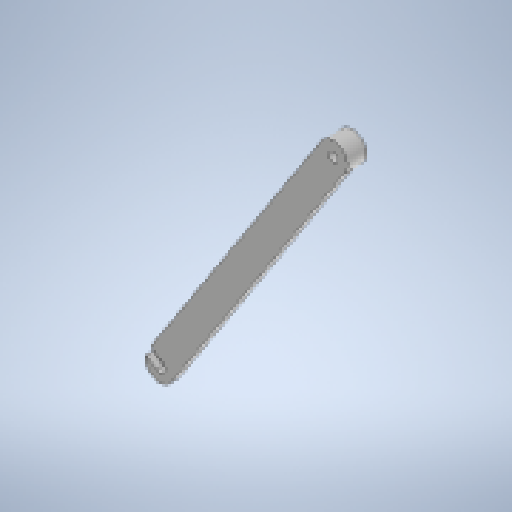
# Autodesk Inventor part: TheHandle
Saved by Autodesk Inventor 2025.1 (Build 291241000, 241)
## iProperties
Created: 2026-05-10
Part Number: TheHandle
Material: Generic
Document SubType Name: Modeling
Designer: User
Density: 1 g/cm^3
Appearance: Default
Author: User
## iProperties of the stored document TheHandle_Left_3DPrint.ipt
Created: 2026-05-12
Part Number: TheHandle_Left_3DPrint
Material: Generic
Document SubType Name: Modeling
Designer: User
Density: 1 g/cm^3
Appearance: Default
Author: User
Autodesk Inventor part; units mm, degrees
ref_plane "YZ Plane" through (0, 0, 0) normal (1, 0, 0) x (0, 1, 0)
ref_plane "XZ Plane" through (0, 0, 0) normal (0, 1, 0) x (-1, 0, 0)
ref_plane "XY Plane" through (0, 0, 0) normal (0, 0, 1) x (1, 0, 0)
sketch "Sketch1" plane through (0, 0, 0) normal (0, 0, 1) x (1, 0, 0)
  circle A0 centre (33.7394, 8.5) radius 2.5 projected
  circle A1 centre (-57.3324, -132.0207) radius 2.5 projected
  circle A2 centre (33.7394, 8.5) radius 7.5
  line L0 (40.0332, 4.421) -> (-51.0386, -136.0997)
  arc A3 (-64.7058, -130.6488) -> (-58.937, -134.5557) centre (33.7394, 8.5) ccw
  line L1 (27.4456, 12.579) -> (-61.9015, -125.2806)
  arc A4 (-64.7058, -130.6488) -> (-51.0386, -136.0997) centre (-57.3324, -132.0207) ccw
  arc A5 (-58.991, -134.5207) -> (-55.7273, -129.486) centre (-57.3324, -132.0207) ccw
  arc A6 (-61.9015, -125.2806) -> (-55.6742, -129.5204) centre (33.7394, 8.5) ccw
  point P0 (0, 0)
  dimension "d1" = 15
  constraints: 14 point on circle, 5 centre point, 4 coincident, 4 end point, 3 tangent
  measures "d1" diameter of A2
extrude "Extrusion1" add sketch "Sketch1" along normal blind 4 contours A2 | A2 L0 A4 A3 A5 A6 L1
sketch "Sketch2" plane through (0, 0, 0) normal (0, 0, -1) x (-1, 0, 0)
  circle A0 centre (-33.7394, 8.5) radius 2.5 projected
  circle A1 centre (-33.7394, 8.5) radius 2.5 projected
  circle A2 centre (-33.7394, 8.5) radius 7.5
  point P0 (0, 0)
  constraints: 1 centre point, 1 coincident
ref_plane "Work Plane1" through (-39.4645, -13.5002, -6.146) normal (0, 0, 1) x (1, 0.0000023, 0)
extrude "Extrusion2" add sketch "Sketch2" along normal up to surface (6.146 mm away)
sketch "Sketch3" plane through (0, 0, 4) normal (0, 0, 1) x (1, 0, 0)
  arc A0 (-64.7058, -130.6488) -> (-51.0386, -136.0997) centre (-57.3324, -132.0207) ccw projected
  arc A1 (-64.7058, -130.6488) -> (-58.991, -134.5207) centre (33.7394, 8.5) ccw projected
  line L0 (-51.0386, -136.0997) -> (40.0332, 4.421) projected
  line L1 (43.3899, 2.2455) -> (-47.6819, -138.2752)
  arc A2 (-66.1549, -124.6441) -> (-47.6819, -138.2752) centre (-57.3324, -132.0207) ccw
  arc A3 (-66.1549, -124.6441) -> (-56.8149, -131.1644) centre (33.7394, 8.5) ccw
  arc A4 (-58.991, -134.5207) -> (-55.7273, -129.486) centre (-57.3324, -132.0207) ccw projected
  arc A5 (-64.7058, -130.6488) -> (-58.991, -134.5207) centre (33.7394, 8.5) ccw projected
  line L2 (-58.991, -134.5207) -> (-64.7058, -130.6488)
  line L3 (-58.991, -134.5207) -> (-68.2061, -128.2773)
  line L4 (48.5795, -33.2403) -> (24.2754, 1.9668)
  line L5 (45.2876, -35.5127) -> (20.9835, -0.3056)
  point P0 (0, 0)
  point P1 (31.6873, -15.8111)
  point P2 (29.2288, -12.2498)
  point P3 (-64.7058, -130.6488)
  dimension "d9" = 4
  dimension "d10" = 4
  constraints: 10 end point, 5 point on circle, 2 centre point, 1 parallel, 1 point on line, 5 other
  measures "d9" distance between parallel lines of L0 L1
  measures "d10" distance between parallel lines of L4 L5
extrude "Extrusion3" add sketch "Sketch3" along normal mid plane 8 contours A0 L0 L5 L1 A2 L3
sketch "Sketch4" plane through (0, 0, 4) normal (0, 0, 1) x (1, 0, 0)
  line L0 (31.6873, -15.8111) -> (29.2288, -12.2498) projected
  line L1 (27.4456, 12.579) -> (-61.9015, -125.2806) projected
  line L2 (29.2288, -12.2498) -> (40.0332, 4.421) projected
  line L3 (31.6873, -15.8111) -> (-47.6819, -138.2752) projected
  line L4 (31.6873, -15.8111) -> (20.0095, 1.1054)
  line L5 (28.3955, -18.0836) -> (16.7177, -1.167)
  line L6 (-51.0386, -136.0997) -> (29.2288, -12.2498) projected
  point P0 (0, 0)
  point P1 (26.8752, -15.8813)
  point P2 (17.6559, -2.5262)
  dimension "d13" = 4
  constraints: 4 end point, 1 parallel, 1 point on line
  measures "d13" distance between parallel lines of L4 L5
extrude "Extrusion4" add sketch "Sketch4" along normal up to surface (4 mm away)
sketch "Sketch5" plane through (0, 0, 0) normal (0, 0, -1) x (-1, 0, 0)
  line L0 (51.0386, -136.0997) -> (-40.0332, 4.421)
  line L1 (-29.2288, -12.2498) -> (-31.6873, -15.8111) projected
  arc A0 (-27.4456, 12.579) -> (-40.0332, 4.421) centre (-33.7394, 8.5) ccw
  line L2 (-31.6873, -15.8111) -> (-42.9295, 11.0274)
  circle A1 centre (-33.7394, 8.5) radius 7.5 projected
  point P0 (0, 0)
  point P1 (-40.657, 5.6023)
  constraints: 4 end point, 2 point on circle, 1 centre point, 1 tangent, 6 other
extrude "Extrusion5" add sketch "Sketch5" against normal up to surface (4 mm away) contours L1 L2 A0 L0
sketch "Sketch6" plane through (33.7394, 8.5, -6.146) normal (0, 0, -1) x (-1, 0, 0)
  line L0 (106.0034, -163.8557) -> (-106.0036, -163.8552)
  line L1 (106.004, 60.4363) -> (-106.003, 60.4368)
  line L2 (0.0005, 60.4366) -> (-28.9075, 60.4367)
  line L3 (0.0005, 60.4366) -> (28.9085, 60.4365)
  circle A0 centre (0.0005, 60.4366) radius 28.908
  line L4 (0.0005, 60.4366) -> (0.0005, 100.4366)
  circle A1 centre (0.0005, 100.4366) radius 2.5
  circle A2 centre (0.0005, 100.4366) radius 7.5
  arc A3 (6.1722, -4.2608) -> (-6.1722, 4.2608) centre (0, 0) ccw
  circle A4 centre (0, 0) radius 7.5
  circle A5 centre (0, 0) radius 7.5 projected
  line L5 (7.5005, 100.4366) -> (7.5, 0)
  line L6 (-7.4995, 100.4366) -> (-7.5, 0)
  point P0 (33.7394, -8.5)
  point P1 (-7.5, 0)
  point P2 (-6.1722, 4.2608)
  point P3 (7.5, 0)
  dimension "d21" = 57.816
  dimension "d18" = 224.292
  dimension "d19" = 28.908
  dimension "d20" = 28.908
  dimension "d22" = 40
  dimension "d23" = 5
  dimension "d24" = 15
  constraints: 14 end point, 6 point on circle, 4 centre point, 4 coincident, 4 tangent, 2 point on line, 1 midpoint, 1 parallel, 1 vertical, 10 other
  measures "d18" distance between parallel lines of L0 L1
  measures "d19" distance of L2.start L2.end
  measures "d20" distance of L2.start L3.end
  measures "d22" distance of L4.start L4.end
  measures "d23" diameter of A1
  measures "d24" diameter of A2
extrude "Extrusion6" add sketch "Sketch6" against normal up to surface (10.146 mm away) contours L5 A0 L6 L1 | L1 L4 A0 L5 | A0 L4 A2 L5 | L5 A3 A4 L6 A0 | L1 L6 A0 L4 | A0 L6 A2 L4 | A2
chamfer "Chamfer1" distance 6 angle 45 3 edges at (40.3714, 4.9977, 0) (31.6126, 1.3079, 0) (26.2394, 9.6089, 0)
chamfer "Chamfer2" distance 6 angle 45 1 edges at (26.2394, 10.7178, 2)
sketch "Sketch7" plane through (0, 0, 4) normal (0, 0, 1) x (1, 0, 0)
  line L0 (45.2389, 108.9366) -> (45.2393, 24.3216)
  line L1 (41.2393, 20.3216) -> (41.2389, 108.9366)
  line L2 (45.2393, 24.3216) -> (41.2393, 20.3216)
  arc A0 (41.2389, 108.9366) -> (26.2389, 108.9366) centre (33.7389, 108.9366) ccw
  arc A1 (45.2389, 108.9366) -> (22.2389, 108.9365) centre (33.7389, 108.9366) ccw
  line L3 (22.2393, 25.7358) -> (22.2389, 108.9365)
  line L4 (26.2393, 22.1725) -> (26.2389, 108.9366)
  line L5 (22.2393, 24.3216) -> (22.2393, 25.7358)
  arc A2 (26.2393, 22.1725) -> (25.9597, 22.0154) centre (33.7394, 8.5) ccw
  arc A3 (25.9597, 22.0154) -> (25.0869, 21.474) centre (33.7394, 8.5) ccw
  line L6 (22.2393, 25.7358) -> (25.9597, 22.0154)
  point P0 (0, 0)
  constraints: 14 end point, 8 point on circle, 4 centre point, 26 other
extrude "Extrusion7" add sketch "Sketch7" along normal mid plane 10
chamfer "Chamfer3" distance 4 angle 45 3 edges at (33.7389, 116.4366, -1) (41.2391, 64.6291, -1) (26.2391, 65.5545, -1)
sketch "Sketch8" plane through (0, 0, 4) normal (0, 0, 1) x (1, 0, 0)
  circle A0 centre (33.7394, 8.5) radius 2.5
  line L0 (31.6873, -15.8111) -> (20.0095, 1.1054) projected
  line L1 (26.8752, -15.8813) -> (17.6559, -2.5262) projected
  line L2 (22.9762, 5.6828) -> (20.0095, 1.1054) projected
  circle A1 centre (33.7394, 8.5) radius 15.5945
  circle A2 centre (33.7394, 8.5) radius 19.5001
  line L3 (22.2389, 108.9365) -> (22.2393, 25.7358) projected
  line L4 (22.2393, 25.7358) -> (22.2393, 24.2481)
  line L5 (22.2393, 25.7358) -> (25.9597, 22.0154) projected
  arc A3 (26.2393, 22.1725) -> (25.9597, 22.0154) centre (33.7394, 8.5) ccw projected
  line L6 (26.2393, 22.1725) -> (26.2389, 108.9366) projected
  line L7 (17.6559, -2.5262) -> (20.0095, 1.1054) projected
  point P0 (0, 0)
  constraints: 2 centre point, 2 coincident, 2 end point, 1 point on circle, 1 vertical, 5 other
extrude "Extrusion8" add sketch "Sketch8" along normal mid plane 8 contours A2 L5 A1 L7 | L4 L5 A2
sketch "Sketch9" plane through (0, 0, 4) normal (0, 0, 1) x (1, 0, 0)
  arc A0 (25.9597, 22.0154) -> (20.0095, 1.1054) centre (33.7394, 8.5) ccw projected
  arc A1 (26.2393, 22.1725) -> (25.9597, 22.0154) centre (33.7394, 8.5) ccw projected
  line L0 (26.2394, 16.7178) -> (26.2393, 22.1725) projected
  line L1 (22.9762, 5.6828) -> (26.2394, 16.7178) projected
  line L2 (22.9762, 5.6828) -> (20.0095, 1.1054) projected
  point P0 (0, 0)
extrude "Extrusion9" add sketch "Sketch9" against normal up to surface (4 mm away)
chamfer "Chamfer4" distance 1 angle 45 1 edges at (24.0995, 23.8756, 9)
sketch "Sketch10" plane through (0, 0, 8) normal (0, 0, 1) x (1, 0, 0)
  arc A0 (-64.7058, -130.6488) -> (-51.0386, -136.0997) centre (-57.3324, -132.0207) ccw projected
  line L0 (26.8752, -15.8813) -> (-51.0386, -136.0997) projected
  arc A1 (-65.1974, -130.5573) -> (-50.619, -136.3716) centre (-57.3324, -132.0207) ccw
  line L1 (-50.619, -136.3716) -> (27.2948, -16.1532)
  line L2 (17.6559, -2.5262) -> (-61.9015, -125.2806) projected
  line L3 (-57.3324, -132.0207) -> (-65.7644, -145.031)
  line L4 (-61.6833, -138.734) -> (-72.2404, -131.892)
  line L5 (-64.7058, -130.6488) -> (-68.2061, -128.2773) projected
  arc A2 (-68.2061, -128.2773) -> (-47.6819, -138.2752) centre (-57.3324, -132.0207) ccw projected
  arc A3 (-61.9015, -125.2806) -> (-55.7273, -129.486) centre (33.7394, 8.5) ccw projected
  circle A4 centre (-57.3324, -132.0207) radius 8
  point P0 (0, 0)
  point P1 (-50.619, -136.3716)
  point P2 (-49.5245, -133.7635)
  point P3 (-68.616, -134.241)
  dimension "d45" = 0.5
  constraints: 6 end point, 3 point on circle, 2 centre point, 1 coincident, 1 concentric, 1 parallel, 1 perpendicular, 1 point on line, 1 tangent, 1 other
  measures "d45" radial gap between concentric circles of A0 A1
extrude "Extrusion10" cut sketch "Sketch10" against normal up to surface (4 mm away) contours A0 L3 A1 A4 L5 | A0 L0 A4 A1 L3 | A4 A1 L4 A2 L5
sketch "Sketch11" plane through (0, 0, 4) normal (0, 0, 1) x (1, 0, 0)
  line L0 (-33.0524, -85.047) -> (-23.748, -70.736) construction
  line L1 (-23.748, -70.736) -> (-14.7241, -76.6029) construction
  line L2 (-14.7241, -76.6029) -> (-24.0284, -90.9139) construction
  line L3 (-24.0284, -90.9139) -> (-33.0524, -85.047) construction
  line L4 (-19.507, -83.9595) -> (-23.4199, -89.9779)
  line L5 (-23.4199, -89.9779) -> (-32.4438, -84.111)
  line L6 (-32.4438, -84.111) -> (-30.9699, -81.844)
  line L7 (-30.9699, -81.844) -> (-23.6645, -86.5937)
  line L8 (-23.6645, -86.5937) -> (-21.2255, -82.8422)
  line L9 (-21.2255, -82.8422) -> (-19.507, -83.9595)
  line L10 (-22.1817, -72.0873) -> (-24.6444, -75.8753)
  line L11 (-24.6444, -75.8753) -> (-22.9406, -76.9831)
  line L12 (-22.9406, -76.9831) -> (-20.6727, -73.4949)
  line L13 (-20.6727, -73.4949) -> (-18.9542, -74.6122)
  line L14 (-18.9542, -74.6122) -> (-21.2221, -78.1003)
  line L15 (-21.2221, -78.1003) -> (-17.339, -80.6249)
  line L16 (-17.339, -80.6249) -> (-18.8034, -82.8772)
  line L17 (-18.8034, -82.8772) -> (-27.8273, -77.0103)
  line L18 (-27.8273, -77.0103) -> (-23.9002, -70.97)
  line L19 (-23.9002, -70.97) -> (-22.1817, -72.0873)
  point P0 (0, 0)
  constraints: 2 other
emboss "Emboss1" sketch "Sketch11" operation cut depth 0.5 direction (0, 0, -1)
equation "\"d25\" = d22"
body "Solid1"
